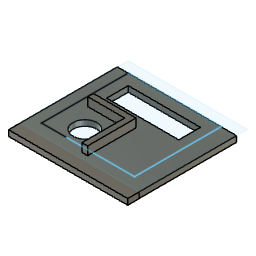
rotary+encoder+holder+plate (Autodesk Fusion 360 design; units mm, degrees)
Autodesk Fusion 360 part; units mm, degrees
sketch "Sketch1" plane through (0, 0, 0) normal (0, 0, 1) x (1, 0, 0)
  line L0 (0, 0) -> (0, 38.1)
  line L1 (0, 38.1) -> (41.91, 38.1)
  line L2 (41.91, 38.1) -> (41.91, 0)
  line L3 (41.91, 0) -> (0, 0)
  dimension "d1" = 38.1
  dimension "d2" = 41.91
  constraint coincident L0.start L3.end
  constraint vertical L0
  constraint perpendicular L0 L1
  constraint perpendicular L1 L2
  constraint perpendicular L0 L3
  measures "d1" distance of L0.start L0.end
  measures "d2" distance of L0.end L1.end
extrude "Extrude1" add sketch "Sketch1" along normal blind 2
sketch "Sketch3" plane through (0, 0, 2) normal (0, 0, 1) x (-1, 0, 0)
  line L0 (-41.91, 0) -> (-41.91, -38.1)
  line L1 (-41.91, -38.1) -> (0, -38.1)
  line L2 (0, -38.1) -> (0, 0)
  line L3 (0, 0) -> (-41.91, 0)
  circle A0 centre (-13.335, -9.525) radius 4.191
  line L4 (-13.335, -9.525) -> (-13.335, -38.1) construction
  line L5 (-13.335, -9.525) -> (-41.91, -9.525) construction
  dimension "d8" = 28.575
  dimension "d9" = 28.575
  dimension "d10" = 8.382
  constraint coincident A0.centre L4.start
  constraint coincident L1 L4.end
  constraint perpendicular L1 L4
  constraint coincident L0 L5.end
  constraint perpendicular L0 L5
  measures "d8" distance of A0.centre L5.end
  measures "d9" distance of A0.centre L4.end
  measures "d10" diameter of A0
extrude "Extrude3" cut sketch "Sketch3" against normal blind 27.94 contours A0
sketch "Sketch4" plane through (0, 0, 2) normal (0, 0, 1) x (-1, 0, 0)
  circle A0 centre (-13.335, -9.525) radius 4.191
  line L0 (-41.91, 0) -> (-41.91, -38.1)
  line L1 (-41.91, -38.1) -> (0, -38.1)
  line L2 (0, -38.1) -> (0, 0)
  line L3 (0, 0) -> (-41.91, 0)
  line L4 (-12.7, -3.81) -> (-3.81, -3.81)
  line L5 (-12.7, -3.81) -> (-36.4901, -3.81)
  line L6 (-3.81, -34.29) -> (-3.81, -3.81)
  line L7 (-3.81, -34.29) -> (-36.4901, -34.29)
  line L8 (-36.4901, -34.29) -> (-36.4901, -3.81)
  dimension "d13" = 3.81
  dimension "d14" = 3.81
  constraint perpendicular L4 L6
  constraint perpendicular L5 L8
  measures "d13" distance of L2 L6
  measures "d14" distance of L3 L4
sketch "Sketch5" plane through (0, 0, 2) normal (0, 0, 1) x (-1, 0, 0)
sketch "Sketch6" plane through (0, 0, 2) normal (0, 0, 1) x (-1, 0, 0)
  line L0 (-13.3454, -9.4898) -> (-13.3454, -1.9898)
  line L1 (-13.3454, -9.4898) -> (-13.3454, -16.9898)
  line L2 (-13.3454, -16.9898) -> (-6.8454, -16.9898)
  line L3 (-13.3454, -16.9898) -> (-19.8454, -16.9898)
  line L4 (-6.8454, -16.9898) -> (-6.8454, -1.9898)
  line L5 (-6.8454, -1.9898) -> (-19.8454, -1.9898)
  line L6 (-19.8454, -16.9898) -> (-19.8454, -1.9898)
  line L7 (-6.8454, -18.9898) -> (-21.8454, -18.9898)
  line L8 (-21.8454, -1.9898) -> (-21.8454, -18.9898)
  line L9 (-19.8454, 0.0102) -> (-21.844, 0.0102)
  line L10 (-21.844, 0.0102) -> (-21.8454, -1.9898)
  line L11 (-19.8454, 0.0102) -> (-4.8454, 0.0102)
  line L12 (-6.8454, -18.9898) -> (-6.8454, -18.796)
  line L13 (-6.8454, -18.9898) -> (-4.8454, -18.9898)
  line L14 (-4.8454, -18.9898) -> (-4.8454, 0.0102)
  line L15 (-19.8454, -1.9898) -> (-20.32, -1.9898)
  line L16 (-20.32, -1.9898) -> (-21.8454, -1.9898)
  line L17 (-6.8454, -16.9898) -> (-6.8454, -18.9898)
  dimension "d15" = 7.5
  dimension "d16" = 7.5
  dimension "d17" = 6.5
  dimension "d18" = 6.5
  dimension "d19" = 15
  dimension "d20" = 13
  dimension "d21" = 2
  dimension "d22" = 2
  dimension "d23" = 2
  dimension "d24" = 2
  constraint parallel L0 L1
  constraint perpendicular L1 L2
  constraint perpendicular L1 L3
  constraint perpendicular L2 L4
  constraint perpendicular L0 L5
  constraint perpendicular L7 L8
  constraint perpendicular L11 L14
  constraint perpendicular L6 L15
  constraint parallel L15 L16
  constraint perpendicular L7 L17
  measures "d15" distance of L0.start L0.end
  measures "d16" distance of L0.start L1.end
  measures "d17" distance of L1.end L2.end
  measures "d18" distance of L1.end L3.end
  measures "d19" distance of L2.end L4.end
  measures "d20" distance of L4.end L5.end
  measures "d21" distance of L2.end L7.start
  measures "d22" distance of L5.end L8.start
  measures "d23" distance of L5.end L9.start
  measures "d24" distance of L7.start L13.end
sketch "Sketch8" plane through (0, 0, 2) normal (0, 0, 1) x (-1, 0, 0)
  line L0 (0, -34.29) -> (-41.91, -34.29)
  line L1 (0, -34.29) -> (0, -38.1)
  line L2 (0, -38.1) -> (-41.91, -38.1)
  line L3 (-41.91, -38.1) -> (-41.91, -34.29)
  constraint horizontal L0
  constraint perpendicular L0 L1
  constraint perpendicular L1 L2
extrude "Extrude4" cut sketch "Sketch8" against normal blind 2.54
sketch "Sketch9" plane through (0, 0, 2) normal (0, 0, 1) x (-1, 0, 0)
  line L0 (0, 0) -> (0, 4)
  line L1 (0, 4) -> (-41.9328, 4)
  line L2 (-41.9328, 4) -> (-41.9328, 0)
  line L3 (-41.9328, 0) -> (0, 0)
  dimension "d27" = 4
  constraint coincident L0.start L3.end
  constraint vertical L0
  constraint perpendicular L0 L1
  constraint perpendicular L1 L2
  constraint perpendicular L0 L3
  measures "d27" distance of L0.start L0.end
extrude "Extrude5" add sketch "Sketch9" against normal blind 2.032
sketch "Sketch10" plane through (0, 0, 2) normal (0, 0, 1) x (-1, 0, 0)
  line L0 (-7.62, -30.48) -> (-33.02, -30.48)
  line L1 (-33.02, -30.48) -> (-33.02, -22.86)
  line L2 (-33.02, -22.86) -> (-7.62, -22.86)
  line L3 (-7.62, -22.86) -> (-7.62, -30.48)
  constraint horizontal L0
  constraint vertical L1
  constraint horizontal L2
  constraint vertical L3
extrude "Extrude6" cut sketch "Sketch10" against normal blind 2.54
extrude "Extrude7" add sketch "Sketch6" along normal blind 3 contours L2 L3 L6 L7 L8 L12 L15 L16 L17
equation "d15 = 15 mm / 2"
equation "d16 = 15 mm / 2"
equation "d17 = 13 mm / 2"
equation "d18 = 13 mm / 2"
